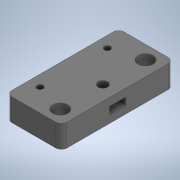
# Autodesk Inventor part: Movingjaw
Saved by Autodesk Inventor 2020.2 (Build 242310000, 310)
## iProperties
Created: 2021-06-22
Part Number: Movingjaw
Material: Generic
Document SubType Name: Modeling
Designer: JK
Density: 1 g/cm^3
Appearance: Gray
Author: JK
Autodesk Inventor part; units mm, degrees
ref_plane "YZ Plane" through (0, 0, 0) normal (1, 0, 0) x (0, 1, 0)
ref_plane "XZ Plane" through (0, 0, 0) normal (0, 1, 0) x (-1, 0, 0)
ref_plane "XY Plane" through (0, 0, 0) normal (0, 0, 1) x (1, 0, 0)
sketch "Sketch1" plane through (0, 0, 0) normal (0, 1, 0) x (-1, 0, 0)
  line L0 (-25, 50) -> (25, 50)
  line L1 (25, 50) -> (25, -50)
  line L2 (25, -50) -> (-25, -50)
  line L3 (-25, -50) -> (-25, 50)
  line L4 (-25, 50) -> (25, -50) construction
  line L5 (25, 50) -> (-25, -50) construction
  circle A0 centre (-11, 38) radius 6.7
  circle A1 centre (-11, -38) radius 6.7
  point P0 (0, 0)
  dimension "d0" = 13.4
  dimension "d1" = 100
  dimension "d2" = 50
  dimension "d4" = 12
  dimension "d5" = 12
  dimension "d6" = 14
  constraints: 12 end point, 2 centre point, 2 midpoint, 2 parallel, 1 equal radius, 1 horizontal, 1 perpendicular, 1 vertical alignment
  measures "d0" diameter of A0
  measures "d1" distance of L0.end L1.end
  measures "d2" distance of L1.end L2.end
  measures "d4" distance from line of L0 A0.centre
  measures "d5" distance from line of L2 A1.centre
  measures "d6" distance from line of L3 A1.centre
extrude "Extrusion1" add sketch "Sketch1" along normal blind 20
sketch "Sketch2" plane through (0, 0, 0) normal (0, -1, 0) x (1, 0, 0)
  circle A0 centre (-15, -30) radius 2.65
  circle A1 centre (-15, 30) radius 2.65
  line L0 (-25, -50) -> (-25, 50) projected
  line L1 (25, -50) -> (-25, -50) projected
  line L2 (-25, 50) -> (25, 50) projected
  point P0 (0, 0)
  dimension "d9" = 5.3
  dimension "d10" = 10
  dimension "d11" = 20
  dimension "d12" = 20
  dimension "d13" = 10
  constraints: 2 centre point, 1 equal radius
  measures "d9" diameter of A0
  measures "d10" distance from line of L0 A0.centre
  measures "d11" distance from line of L1 A0.centre
  measures "d12" distance from line of L2 A1.centre
  measures "d13" distance from line of L0 A1.centre
extrude "Extrusion2" cut sketch "Sketch2" against normal through all
sketch "Sketch3" plane through (0, 0, 0) normal (0, -1, 0) x (1, 0, 0)
  line L0 (25, 50) -> (25, -50) projected
  line L1 (-25, 50) -> (25, 50) projected
  line L2 (25, -50) -> (24, -50)
  line L3 (24, -50) -> (24, 50)
  line L4 (24, 50) -> (25, 50)
  line L5 (25, 50) -> (25, -50)
  point P0 (0, 0)
  dimension "d16" = 1
  constraints: 8 end point, 2 parallel, 1 horizontal, 1 perpendicular, 1 point on line
  measures "d16" distance between parallel lines of L3 L0
extrude "Extrusion3" cut sketch "Sketch3" against normal through all
fillet "Fillet1" radius 5 2 edges at (-25, 10, 50) (-25, 10, -50)
sketch "Sketch4" plane through (0, 0, 0) normal (0, -1, 0) x (1, 0, 0)
  circle A0 centre (-15, -30) radius 2.65 projected
  circle A1 centre (-15, -30) radius 4.1
  circle A2 centre (-15, 30) radius 2.65 projected
  circle A3 centre (-15, 30) radius 4.1
  line L0 (-19.7343, -30) -> (-17.3671, -25.9)
  line L1 (-17.3671, -25.9) -> (-12.6329, -25.9)
  line L2 (-12.6329, -25.9) -> (-10.2657, -30)
  line L3 (-10.2657, -30) -> (-12.6329, -34.1)
  line L4 (-12.6329, -34.1) -> (-17.3671, -34.1)
  line L5 (-17.3671, -34.1) -> (-19.7343, -30)
  line L6 (-19.7311, 29.8275) -> (-17.5149, 34.011)
  line L7 (-17.5149, 34.011) -> (-12.7838, 34.1835)
  line L8 (-12.7838, 34.1835) -> (-10.2689, 30.1725)
  line L9 (-10.2689, 30.1725) -> (-12.4851, 25.989)
  line L10 (-12.4851, 25.989) -> (-17.2162, 25.8165)
  line L11 (-17.2162, 25.8165) -> (-19.7311, 29.8275)
  point P0 (0, 0)
  dimension "d20" = 8.2
  dimension "d21" = 8.2
  constraints: 24 end point, 4 coincident, 2 centre point, 2 tangent, 1 horizontal alignment, 26 other
  measures "d20" diameter of A1
  measures "d21" diameter of A3
extrude "Extrusion4" [suppressed]
sketch "Sketch5" plane through (0, 0, 0) normal (0, -1, 0) x (1, 0, 0)
  circle A0 centre (11, 0) radius 4.15
  circle A1 centre (11, -38) radius 6.7 projected
  point P0 (0, 0)
  dimension "d24" = 8.3
  constraints: 1 centre point, 1 vertical alignment
  measures "d24" diameter of A0
extrude "Extrusion5" cut sketch "Sketch5" against normal through all contours A0
sketch "Sketch6" plane through (24, 0, 50) normal (1, 0, 0) x (0, 0, -1)
  line L0 (57.05, 6.9) -> (42.95, 6.9)
  line L1 (42.95, 6.9) -> (42.95, 13.1)
  line L2 (42.95, 13.1) -> (57.05, 13.1)
  line L3 (57.05, 13.1) -> (57.05, 6.9)
  line L4 (57.05, 6.9) -> (42.95, 13.1) construction
  line L5 (42.95, 6.9) -> (57.05, 13.1) construction
  line L6 (0, 20) -> (100, 20) projected
  point P0 (50, 0)
  point P1 (50, 10)
  dimension "d27" = 10
  dimension "d28" = 14.1
  dimension "d29" = 6.2
  constraints: 12 end point, 2 midpoint, 2 parallel, 1 horizontal, 1 perpendicular
  measures "d27" distance from line of L6 point (50, 10)
  measures "d28" distance between parallel lines of L1 L3
  measures "d29" distance of L2.end L0.start
extrude "Extrusion6" cut sketch "Sketch6" against normal blind 22
fillet "Fillet2" radius 5 2 edges at (24, 10, -50) (24, 10, 50)
sketch "Sketch7" plane through (0, 0, 0) normal (0, -1, 0) x (1, 0, 0)
  circle A0 centre (-15, -30) radius 2.65 projected
  circle A1 centre (-15, -30) radius 4.5
  circle A2 centre (-15, 30) radius 2.65 projected
  circle A3 centre (-15, 30) radius 4.5
  point P0 (0, 0)
  dimension "d35" = 9
  constraints: 2 centre point, 2 coincident, 1 equal radius
  measures "d35" diameter of A1
extrude "Extrusion7" cut sketch "Sketch7" against normal blind 5 contours A1 | A2 | A3
body "Solid1"
